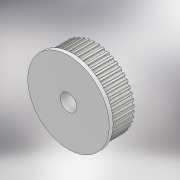
# Autodesk Inventor part: GT2Shaft48T
Saved by Autodesk Inventor 2018.2 (Build 222227000, 227)
## iProperties
Created: 2018-02-13
Part Number: GT2Shaft48T
Material: ABS Plastic
Document SubType Name: Modeling
Designer: Moochster
Density: 1.06 g/cm^3
Appearance: Smooth - White
Mass: 0.74321 g
Surface Area: 11.7432 cm^2
Volume: 0.701142 cm^3
Author: Moochster
Autodesk Inventor part; units mm, degrees
ref_plane "YZ Plane" through (0, 0, 0) normal (1, 0, 0) x (0, 1, 0)
ref_plane "XZ Plane" through (0, 0, 0) normal (0, 1, 0) x (-1, 0, 0)
ref_plane "XY Plane" through (0, 0, 0) normal (0, 0, 1) x (1, 0, 0)
sketch "Sketch1" plane through (0, 0, 0) normal (0, 1, 0) x (-1, 0, 0)
  circle A0 centre (0, 0) radius 3.175
  circle A1 centre (0, 0) radius 14.7441
  dimension "BoreD" = 6.35
  dimension "OuterD" = 29.4882
  constraints: 2 centre point, 2 coincident
  measures "BoreD" diameter of A0
  measures "OuterD" diameter of A1
extrude "Extrusion1" add sketch "Sketch1" along normal blind 9
sketch "Sketch2" plane through (0, 0, 0) normal (0, -1, 0) x (1, 0, 0)
  circle A0 centre (0, 0) radius 14.7441 projected
  arc A1 (0.4956, -14.5601) -> (0.6509, -14.7297) centre (0.6443, -14.5799) ccw
  arc A2 (0.4956, -14.5601) -> (-0.4956, -14.5601) centre (0, -14.4941) ccw
  arc A3 (-0.6509, -14.7297) -> (-0.4956, -14.5601) centre (-0.6443, -14.5799) ccw
  point P0 (0, -14.7441)
  dimension "d9" = 0.5
  dimension "d10" = 0.15
  dimension "Depth" = 0.25
  constraints: 9 point on circle, 4 tangent, 3 centre point, 2 vertical alignment, 1 equal radius
  measures "d9" radius of A2
  measures "d10" radius of A3
  measures "Depth" distance of point (0, -14.744) A2.centre
extrude "Extrusion2" cut sketch "Sketch2" against normal up to next contours A3 A2 A1 A0 picked at (0, -14.493)
pattern_circular "Circular Pattern1" count 48 over 360 about axis through (0, -10, 0) along (0, 1, 0) of "Extrusion2"
sketch "Sketch3" plane through (0, 0, 0) normal (0, -1, 0) x (1, 0, 0)
  circle A0 centre (0, 0) radius 15.6191
  circle A1 centre (0, 0) radius 3.175
  dimension "FaceD" = 31.2382
  dimension "d18" = 6.35
  constraints: 2 centre point, 2 coincident
  measures "FaceD" diameter of A0
  measures "d18" diameter of A1
extrude "Extrusion3" add sketch "Sketch3" along normal blind 1.5
sketch "Sketch4" plane through (0, 9, 0) normal (0, 1, 0) x (1, 0, 0)
  circle A0 centre (0, 0) radius 3.175 projected
  circle A1 centre (0, 0) radius 5.175
  circle A2 centre (0, 0) radius 15.6191 projected
  dimension "d21" = 2
  constraints: 1 centre point, 1 coincident
  measures "d21" radial gap between concentric circles of A0 A1
extrude "Extrusion4" [suppressed]
extrude "Extrusion5" add sketch "Sketch4" along normal blind 6 contours A1
sketch "Sketch5" plane through (0, 0, 0) normal (1, 0, 0) x (0, 1, 0)
  circle A0 centre (12, 0) radius 1.5
  line L0 (9, -5.175) -> (15, -5.175) projected
  point P0 (0, 0)
  point P1 (12, -5.175)
  dimension "d26" = 3
  constraints: 1 centre point, 1 horizontal alignment, 1 midpoint, 1 vertical alignment
  measures "d26" diameter of A0
extrude "Extrusion6" cut sketch "Sketch5" along normal through all both and the other way through all
equation "\"OuterD\" = 0.614338 * Teeth"
equation "\"Depth\" = Pitch"
equation "\"d18\" = BoreD"
equation "\"BeltWidth\" = 8"
equation "\"Pitch\" = 0.25"
equation "\"Teeth\" = 48"
body "Solid1"
